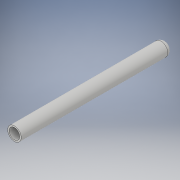
# Autodesk Inventor part: A
Saved by Autodesk Inventor 2017 (Build 210142000, 142)
## iProperties
Part Number: A
Material: 一般
Document SubType Name: Modeling
Designer: user
Density: 1 g/cm^3
Appearance: 預設
Author: user
Autodesk Inventor part; units mm, degrees
ref_plane "YZ Plane" through (0, 0, 0) normal (1, 0, 0) x (0, 1, 0)
ref_plane "XZ Plane" through (0, 0, 0) normal (0, 1, 0) x (-1, 0, 0)
ref_plane "XY Plane" through (0, 0, 0) normal (0, 0, 1) x (1, 0, 0)
sketch "草圖1" plane through (0, 0, 0) normal (1, 0, 0) x (0, 1, 0)
  line L0 (0, 0) -> (4.5, 0)
  line L1 (4.5, 0) -> (4.5, -100)
  line L2 (4.5, -100) -> (0, -100)
  line L3 (0, -100) -> (0, 0)
  dimension "d3" = 100
  dimension "d4" = 4.5
  constraints: 8 end point, 2 parallel, 1 horizontal, 1 perpendicular
  measures "d3" distance of L2.end L0.start
  measures "d4" distance of L1.end L2.end
revolve "迴轉1" add sketch "草圖1" angle 360 about axis through (0, 0, -100) along (0, 0, 1)
shell "薄殼2" thickness 1 removed faces 1 at (-1.8702, -1.7271, 0)
fillet "圓角3" radius 3 1 edges at (0, -3.5, -99)
fillet "圓角4" radius 3 1 edges at (0, -4.5, -100)
